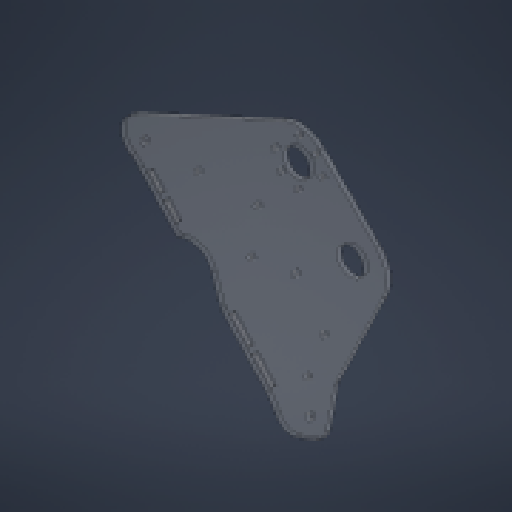
# Autodesk Inventor part: 4Bar_Input Side
Saved by Autodesk Inventor 2026 (Build 300175000, 175)
## iProperties
Created: 2026-01-17
Part Number: 4Bar_Input Side
Material: Polycarbonate, Clear
Document SubType Name: Modeling
Designer: 110
Density: 1.2 g/cm^3
Appearance: Polycarbonate - Clear
Mass: 252.928 g
Surface Area: 948.68 cm^2
Volume: 210.773 cm^3
Author: 110
Autodesk Inventor part; units mm, degrees
ref_plane "YZ Plane" through (0, 0, 0) normal (1, 0, 0) x (0, 1, 0)
ref_plane "XZ Plane" through (0, 0, 0) normal (0, 1, 0) x (-1, 0, 0)
ref_plane "XY Plane" through (0, 0, 0) normal (0, 0, 1) x (1, 0, 0)
sketch "Sketch1" plane through (0, 0, 0) normal (0, 0, 1) x (1, 0, 0)
  arc A0 (-9.3696, 20.3364) -> (-12.3686, -18.6649) centre (0, 0) ccw
  circle A1 centre (222.25, 0) radius 38.1 construction
  arc A2 (256.5122, -16.6647) -> (249.2444, 26.8871) centre (222.25, 0) ccw
  arc A3 (141.7475, -180.5258) -> (173.705, -185.472) centre (159.267, -173.0444) ccw
  line L0 (0, 0) -> (203.2, 0) construction
  line L1 (222.25, 0) -> (159.267, -173.0444) construction
  line L2 (0, 160.1612) -> (0, -260.5824) construction
  line L3 (-102.1099, 0) -> (329.65, 0) construction
  line L4 (0, 0) -> (222.25, 0) construction
  circle A4 centre (187.8917, -94.3987) radius 75.057 construction
  circle A5 centre (222.25, 0) radius 25.4 construction
  circle A6 centre (159.267, -173.0444) radius 19.05 construction
  circle A7 centre (164.8344, 62.1438) radius 25.4 construction
  arc A8 (189.5792, 86.7903) -> (150.2199, 93.8641) centre (164.8344, 62.1438) ccw
  line L5 (189.5792, 86.7903) -> (249.2444, 26.8871)
  line L6 (150.2199, 93.8641) -> (-9.3696, 20.3364)
  line L7 (222.25, 0) -> (164.8344, 62.1438) construction
  circle A9 centre (222.25, 0) radius 45.72 construction
  arc A10 (74.4836, -84.1243) -> (39.1965, -69.0126) centre (50.2908, -91.8616) ccw
  line L8 (50.2908, -91.8616) -> (-18.6562, -17.2368) construction
  line L9 (-18.6562, -17.2368) -> (0, 0) construction
  line L10 (132.3414, -166.0026) -> (84.8578, -114.6087)
  line L11 (35.4777, -68.3111) -> (-3.1175, -26.5376)
  arc A11 (35.4777, -68.3111) -> (39.1965, -69.0126) centre (37.8097, -66.1565) ccw
  arc A12 (-3.1175, -26.5376) -> (-12.3686, -18.6649) centre (-40.4299, -61.0111) ccw
  arc A13 (141.7475, -180.5258) -> (132.3414, -166.0026) centre (95.029, -200.4761) ccw
  line L12 (74.4836, -84.1243) -> (83.4737, -112.2339)
  line L13 (135.6596, -160.2741) -> (92.5677, -113.6336)
  line L14 (92.5677, -113.6336) -> (94.9184, -111.4618)
  line L15 (94.9184, -111.4618) -> (138.0102, -158.1023)
  line L16 (138.0102, -158.1023) -> (135.6596, -160.2741)
  line L17 (135.6596, -160.2741) -> (94.9184, -111.4618) construction
  line L18 (92.5677, -113.6336) -> (138.0102, -158.1023) construction
  line L19 (116.2682, -139.2859) -> (118.6189, -137.1141)
  line L20 (118.6189, -137.1141) -> (114.3097, -132.45)
  line L21 (114.3097, -132.45) -> (111.959, -134.6219)
  line L22 (111.959, -134.6219) -> (116.2682, -139.2859)
  line L23 (116.2682, -139.2859) -> (114.3097, -132.45) construction
  line L24 (118.6189, -137.1141) -> (111.959, -134.6219) construction
  line L25 (35.0013, -58.4382) -> (4.837, -25.7898)
  line L26 (4.837, -25.7898) -> (7.1877, -23.618)
  line L27 (7.1877, -23.618) -> (37.352, -56.2664)
  line L28 (37.352, -56.2664) -> (35.0013, -58.4382)
  line L29 (35.0013, -58.4382) -> (7.1877, -23.618) construction
  line L30 (4.837, -25.7898) -> (37.352, -56.2664) construction
  line L31 (0, 0) -> (30.1643, -32.6484) construction
  line L32 (30.1643, -32.6484) -> (21.0945, -41.0281) construction
  line L33 (24.4244, -42.2742) -> (20.1153, -37.6102)
  line L34 (20.1153, -37.6102) -> (17.7646, -39.782)
  line L35 (17.7646, -39.782) -> (22.0738, -44.4461)
  line L36 (22.0738, -44.4461) -> (24.4244, -42.2742)
  line L37 (24.4244, -42.2742) -> (17.7646, -39.782) construction
  line L38 (20.1153, -37.6102) -> (22.0738, -44.4461) construction
  arc A14 (83.4737, -112.2339) -> (84.8578, -114.6087) centre (89.5219, -110.2996) ccw
  circle A15 centre (177.2487, -166.7545) radius 19.05 construction
  line L39 (165.5568, -191.0261) -> (183.5385, -184.7362)
  arc A16 (183.5385, -184.7362) -> (195.9526, -170.3691) centre (177.2487, -166.7545) ccw
  line L40 (195.9526, -170.3691) -> (204.9972, -123.5672)
  line L41 (256.5122, -16.6647) -> (206.0458, -120.422)
  arc A17 (206.0458, -120.422) -> (204.9972, -123.5672) centre (217.4665, -125.9769) ccw
  point P0 (165.7825, -155.1433)
  point P1 (191.2238, 33.5812)
  point P2 (-1.8157, -27.9466)
  point P3 (83.9025, -113.5748)
  point P4 (115.289, -135.868)
  point P5 (111.959, -134.6219)
  point P6 (114.3097, -132.45)
  point P7 (116.2682, -139.2859)
  point P8 (118.6189, -137.1141)
  dimension "d30" = 76.2
  dimension "d110" = 91.44
  dimension "d31" = 44.7822
  dimension "d34" = 184.15
  dimension "d39" = 19.05
  dimension "d80" = 22.3911
  dimension "d86" = 222.25
  dimension "d87" = 0
  dimension "d101" = 70
  dimension "d102" = 150.114
  dimension "d103" = 50.8
  dimension "d104" = 38.1
  dimension "d107" = 84.6074
  dimension "d108" = 75.2075
  dimension "d109" = 34.925
  dimension "d139" = 50.8
  dimension "d140" = 25.4
  dimension "d141" = 101.6
  dimension "d142" = 178.689
  dimension "d143" = 3.175
  dimension "d144" = 155
  dimension "d148" = 63.5
  dimension "d149" = 25.4
  dimension "d152" = 6.35
  dimension "d153" = 3.2004
  dimension "d154" = 6.35
  dimension "d155" = 173.99
  dimension "d156" = 44.45
  dimension "d157" = 44.45
  dimension "d158" = 169.164
  dimension "d159" = 3.2004
  dimension "d160" = 6.35
  dimension "d161" = 50.8
  dimension "d162" = 6.35
  dimension "d163" = 172.72
  dimension "d164" = 38.1
  dimension "d166" = 165
  dimension "d167" = 12.7
  constraints: 80 end point, 30 point on circle, 20 tangent, 16 centre point, 14 parallel, 12 coincident, 8 midpoint, 8 perpendicular, 8 point on line, 3 collinear, 2 equal radius, 1 concentric, 8 other
  measures "d31" diameter of A0
  measures "d34" distance of L1.start L1.end
  measures "d39" radius of A3
  measures "d80" radius of A0
  measures "d86" distance of L0.start L1.start
  measures "d87" distance between parallel lines of L4 L0
  measures "d101" angle of L0 L1
  measures "d102" diameter of A4
  measures "d103" diameter of A5
  measures "d104" diameter of A6
  measures "d107" distance of point (164.834, 62.144) L1.start
  measures "d108" distance from line of point (164.834, 62.144) L1
  measures "d109" radius of A8
  measures "d139" diameter of A10
  measures "d140" distance of L8.end L0.start
  measures "d141" distance of L8.start L8.end
  measures "d142" distance from line of point (164.834, 62.144) L10
  measures "d143" radius of A11
  measures "d144" angle of L10 L12
  measures "d148" distance of L14.end L15.end
  measures "d149" distance from line of L1.end L16
  measures "d152" distance of L20.end L19.end
  measures "d153" distance of L25.end L26.end
  measures "d154" distance between parallel lines of L25 L11
  measures "d155" distance from line of point (164.834, 62.144) L27
  measures "d156" distance of L26.end L27.end
  measures "d157" distance of L0.start L31.end
  measures "d158" distance from line of L1.start L15
  measures "d159" distance of L13.end L14.end
  measures "d160" distance of L33.start L33.end
  measures "d161" radius of A13
  measures "d162" radius of A14
  measures "d163" distance of point (222.25, 0) point (177.249, -166.755)
  measures "d164" diameter of A15
  measures "d166" angle of L41 L40
  measures "d167" radius of A17
extrude "Extrusion1" add sketch "Sketch1" along normal blind 4.7625 contours L6 A8 L5 A2 L41 A17 L40 A16 L39 A3 A13 L10 A14 L12 A10 A11 L11 A12 A0 | L13 L21 L15 L19 | L25 L34 L27 L36
sketch "Sketch2" plane through (0, 0, 4.7625) normal (0, 0, 1) x (1, 0, 0)
  arc A0 (141.7475, -180.5258) -> (165.5568, -191.0261) centre (159.267, -173.0444) ccw projected
  arc A1 (-9.3696, 20.3364) -> (-12.3686, -18.6649) centre (0, 0) ccw projected
  line L0 (206.0458, -120.422) -> (256.5122, -16.6647) projected
  arc A2 (256.5122, -16.6647) -> (249.2444, 26.8871) centre (222.25, 0) ccw projected
  line L1 (150.2199, 93.8641) -> (-9.3696, 20.3364) projected
  line L2 (249.2444, 26.8871) -> (189.5792, 86.7903) projected
  arc A3 (189.5792, 86.7903) -> (150.2199, 93.8641) centre (164.8344, 62.1438) ccw projected
  line L3 (-3.1175, -26.5376) -> (35.4777, -68.3111) projected
  arc A4 (74.4836, -84.1243) -> (39.1965, -69.0126) centre (50.2908, -91.8616) ccw projected
  line L4 (84.8578, -114.6087) -> (132.3414, -166.0026) projected
  arc A5 (-3.1175, -26.5376) -> (-12.3686, -18.6649) centre (-40.4299, -61.0111) ccw projected
  arc A6 (35.4777, -68.3111) -> (39.1965, -69.0126) centre (37.8097, -66.1565) ccw projected
  arc A7 (141.7475, -180.5258) -> (132.3414, -166.0026) centre (95.029, -200.4761) ccw projected
  line L5 (74.4836, -84.1243) -> (83.4737, -112.2339) projected
  arc A8 (83.4737, -112.2339) -> (84.8578, -114.6087) centre (89.5219, -110.2996) ccw projected
  line L6 (165.5568, -191.0261) -> (183.5385, -184.7362) projected
  arc A9 (183.5385, -184.7362) -> (195.9526, -170.3691) centre (177.2487, -166.7545) ccw projected
  line L7 (195.9526, -170.3691) -> (204.9972, -123.5672) projected
  arc A10 (206.0458, -120.422) -> (204.9972, -123.5672) centre (217.4665, -125.9769) ccw projected
  constraints: 1 coincident
hole "Structure Holes" at (0, 0, 4.7625) at (177.2487, -166.7545, 4.7625) direction (0, 0, -1) diameter 6.35 end through all
sketch "Sketch4" plane through (0, 0, 4.7625) normal (0, 0, 1) x (1, 0, 0)
  arc A0 (141.7475, -180.5258) -> (165.5568, -191.0261) centre (159.267, -173.0444) ccw projected
  arc A1 (-9.3696, 20.3364) -> (-12.3686, -18.6649) centre (0, 0) ccw projected
  line L0 (206.0458, -120.422) -> (256.5122, -16.6647) projected
  arc A2 (256.5122, -16.6647) -> (249.2444, 26.8871) centre (222.25, 0) ccw projected
  line L1 (0, 0) -> (114.3, -50.8) construction
  line L2 (150.2199, 93.8641) -> (-9.3696, 20.3364) projected
  line L3 (249.2444, 26.8871) -> (189.5792, 86.7903) projected
  arc A3 (189.5792, 86.7903) -> (150.2199, 93.8641) centre (164.8344, 62.1438) ccw projected
  line L4 (164.8344, 62.1438) -> (256.9422, -37.5491) construction
  line L5 (-3.1175, -26.5376) -> (35.4777, -68.3111) projected
  arc A4 (74.4836, -84.1243) -> (39.1965, -69.0126) centre (50.2908, -91.8616) ccw projected
  line L6 (84.8578, -114.6087) -> (132.3414, -166.0026) projected
  arc A5 (-3.1175, -26.5376) -> (-12.3686, -18.6649) centre (-40.4299, -61.0111) ccw projected
  arc A6 (35.4777, -68.3111) -> (39.1965, -69.0126) centre (37.8097, -66.1565) ccw projected
  arc A7 (141.7475, -180.5258) -> (132.3414, -166.0026) centre (95.029, -200.4761) ccw projected
  line L7 (74.4836, -84.1243) -> (83.4737, -112.2339) projected
  arc A8 (83.4737, -112.2339) -> (84.8578, -114.6087) centre (89.5219, -110.2996) ccw projected
  line L8 (165.5568, -191.0261) -> (183.5385, -184.7362) projected
  arc A9 (183.5385, -184.7362) -> (195.9526, -170.3691) centre (177.2487, -166.7545) ccw projected
  line L9 (195.9526, -170.3691) -> (204.9972, -123.5672) projected
  arc A10 (206.0458, -120.422) -> (204.9972, -123.5672) centre (217.4665, -125.9769) ccw projected
  point P0 (139.4542, 63.1476)
  point P1 (146.1782, 44.9071)
  point P2 (163.8307, 36.7637)
  point P3 (182.0711, 43.4876)
  point P4 (190.2145, 61.1401)
  point P5 (183.4906, 79.3806)
  point P6 (165.8381, 87.524)
  point P7 (147.5976, 80.8001)
  dimension "d83" = 114.3
  dimension "d84" = 50.8
  dimension "d132" = 25.4
  dimension "d135" = 360
  constraints: 4 end point, 3 coincident, 1 point on line, 9 other
  measures "d83" horizontal distance of L1.start L1.end
  measures "d84" vertical distance of L1.start L1.end
  measures "d132" distance of L4.start point (139.454, 63.148)
hole "BearingHole" at (222.25, 0, 4.7625) at (164.8344, 62.1438, 4.7625) direction (0, 0, -1) diameter 28.575 end through all
hole "Hole4" at (114.3, -50.8, 4.7625) direction (0, 0, -1) diameter 5.1054 end through all clearance for "Socket Head Cap Screw" size "#10" standard "Ansi Unified Screw Threads"
sketch "Sketch3" plane through (0, 0, 0) normal (0, 0, -1) x (-1, 0, 0)
  line L0 (0, 0) -> (-222.25, 0) construction
  line L1 (-222.25, 0) -> (-159.267, -173.0444) construction
  line L2 (-84.8185, 0) -> (-175.2456, -129.1434) construction
  line L3 (-130.032, -64.5717) -> (-161.2417, -42.7184) construction
  point P0 (-184.15, 0)
  point P1 (-120.65, 0)
  point P2 (-57.15, 0)
  point P3 (-209.219, -35.8023)
  point P4 (-191.8444, -83.5387)
  point P5 (-174.4698, -131.2751)
  dimension "d10" = 137.4315
  dimension "d11" = 137.4315
  dimension "d12" = 38.1
  dimension "d43" = 38.1
  dimension "d46" = 63.5
  dimension "d51" = 38.1
  dimension "d54" = 50.8
  constraints: 8 end point, 4 point on line, 2 coincident, 1 horizontal, 1 midpoint, 1 perpendicular, 5 other
  measures "d10" distance of L0.end L2.end
  measures "d11" distance of L0.end L2.start
  measures "d12" distance of L3.start L3.end
  measures "d43" distance of point (-184.15, 0) L0.end
  measures "d46" distance of point (-184.15, 0) point (-120.65, 0)
  measures "d51" distance of point (-209.219, -35.802) L0.end
  measures "d54" distance of point (-209.219, -35.802) point (-191.844, -83.539)
ref_plane "Inner Pitch Plane" through (0, 0, 0) normal (1, 0, 0) x (0, 1, 0)
hole "Hole6" at (165.8381, 87.524, 4.7625) at (183.4906, 79.3806, 4.7625) at (190.2145, 61.1401, 4.7625) at (163.8307, 36.7637, 4.7625) at (146.1782, 44.9071, 4.7625) at (139.4542, 63.1476, 4.7625) direction (0, 0, -1) diameter 4.9784 end through all clearance for "Flat Head Machine Screw (82)" size "#10" standard "Ansi Unified Screw Threads"
hole "Hole8" at (161.2417, -42.7184, 0) at (0, 0, 0) at (222.25, 0, 0) at (120.65, 0, 0) at (57.15, 0, 0) at (191.8444, -83.5387, 0) at (174.4698, -131.2751, 0) direction (0, 0, 1) diameter 5.1054 end through all clearance for "Flat Head Machine Screw (82)" size "#10" standard "Ansi Unified Screw Threads"
equation "\"d10\" = d11"
equation "\"d51\" = d43"
body "Solid1"
